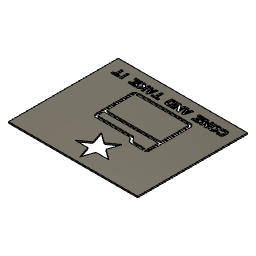
ComeAndTakeIt (Autodesk Fusion 360 design; units mm, degrees)
Autodesk Fusion 360 part; units mm, degrees
(part 1 of 2)
sketch "Sketch1" plane through (0, 0, 0) normal (0, 1, 0) x (1, 0, 0)
  line L0 (0, 0) -> (140, 0)
  line L1 (140, 0) -> (140, -85)
  line L2 (140, -85) -> (0, -85)
  line L3 (0, -85) -> (0, 0)
  constraint horizontal L0
  constraint vertical L1
  constraint horizontal L2
  constraint vertical L3
  constraint coincident L0.start L3.end
extrude "Extrude1" add sketch "Sketch1" along normal blind 2
sketch "Sketch2" plane through (0, 2, 0) normal (0, 1, 0) x (-1, 0, 0)
  line L0 (0, 85) -> (-140, 85)
  line L1 (-140, 85) -> (-140, 0)
  line L2 (-140, 0) -> (0, 0)
  line L3 (0, 0) -> (0, 85)
  spline S0 degree 3 poles (-116.9301, 6.5861) (-117.7721, 6.8255) (-117.8476, 7.0711) (-117.8471, 9.57) knots 0 0 0 0 1 1 1 1
  spline S1 degree 3 poles (-117.8471, 9.57) (-117.8467, 12.3494) (-117.7458, 12.5338) (-116.1845, 12.6085) knots 0 0 0 0 1 1 1 1
  line L4 (-116.1845, 12.6085) -> (-115.3705, 12.6474)
  line L5 (-115.3705, 12.6474) -> (-115.3705, 11.8564)
  line L6 (-115.3705, 11.8564) -> (-115.3705, 11.0653)
  line L7 (-115.3705, 11.0653) -> (-115.8292, 11.0653)
  line L8 (-115.8292, 11.0653) -> (-116.2879, 11.0653)
  line L9 (-116.2879, 11.0653) -> (-116.2879, 9.5516)
  line L10 (-116.2879, 9.5516) -> (-116.2879, 8.0379)
  line L11 (-116.2879, 8.0379) -> (-115.8292, 8.0379)
  line L12 (-115.8292, 8.0379) -> (-115.3705, 8.0379)
  line L13 (-115.3705, 8.0379) -> (-115.3705, 7.2581)
  line L14 (-115.3705, 7.2581) -> (-115.3705, 6.4783)
  line L15 (-115.3705, 6.4783) -> (-115.9897, 6.4865)
  spline S2 degree 3 poles (-115.9897, 6.4865) (-116.3303, 6.4911) (-116.7535, 6.5359) (-116.9301, 6.5861) knots 0 0 0 0 1 1 1 1
  line L16 (-115.0035, 7.2486) -> (-115.0035, 8.0379)
  line L17 (-115.0035, 8.0379) -> (-114.5448, 8.0379)
  spline S3 degree 3 poles (-114.5448, 8.0379) (-114.1167, 8.0379) (-114.0861, 8.0532) (-114.0861, 8.2672) knots 0 0 0 0 1 1 1 1
  spline S4 degree 3 poles (-114.0861, 8.2672) (-114.0861, 8.4941) (-114.0776, 8.4966) (-113.2956, 8.4966) knots 0 0 0 0 1 1 1 1
  line L18 (-113.2956, 8.4966) -> (-112.5051, 8.4966)
  line L19 (-112.5051, 8.4966) -> (-112.543, 7.9012)
  spline S5 degree 3 poles (-112.543, 7.9012) (-112.6079, 6.8826) (-113.0093, 6.551) (-114.2466, 6.4942) knots 0 0 0 0 1 1 1 1
  line L20 (-114.2466, 6.4942) -> (-115.0035, 6.4594)
  line L21 (-115.0035, 6.4594) -> (-115.0035, 7.2486)
  spline S6 degree 3 poles (-110.7834, 6.5861) (-111.6154, 6.8226) (-111.7009, 7.1053) (-111.7005, 9.6175) knots 0 0 0 0 1 1 1 1
  spline S7 degree 3 poles (-111.7005, 9.6175) (-111.7, 12.3429) (-111.5937, 12.5341) (-110.0378, 12.6085) knots 0 0 0 0 1 1 1 1
  line L22 (-110.0378, 12.6085) -> (-109.2238, 12.6474)
  line L23 (-109.2238, 12.6474) -> (-109.2238, 11.8564)
  line L24 (-109.2238, 11.8564) -> (-109.2238, 11.0653)
  line L25 (-109.2238, 11.0653) -> (-109.6825, 11.0653)
  line L26 (-109.6825, 11.0653) -> (-110.1412, 11.0653)
  line L27 (-110.1412, 11.0653) -> (-110.1412, 9.5516)
  line L28 (-110.1412, 9.5516) -> (-110.1412, 8.0379)
  line L29 (-110.1412, 8.0379) -> (-109.6825, 8.0379)
  line L30 (-109.6825, 8.0379) -> (-109.2238, 8.0379)
  line L31 (-109.2238, 8.0379) -> (-109.2238, 7.2581)
  line L32 (-109.2238, 7.2581) -> (-109.2238, 6.4783)
  line L33 (-109.2238, 6.4783) -> (-109.843, 6.4865)
  spline S8 degree 3 poles (-109.843, 6.4865) (-110.1836, 6.4911) (-110.6068, 6.5359) (-110.7834, 6.5861) knots 0 0 0 0 1 1 1 1
  line L34 (-108.8568, 7.2486) -> (-108.8568, 8.0379)
  line L35 (-108.8568, 8.0379) -> (-108.3981, 8.0379)
  line L36 (-108.3981, 8.0379) -> (-107.9394, 8.0379)
  line L37 (-107.9394, 8.0379) -> (-107.9394, 9.5516)
  line L38 (-107.9394, 9.5516) -> (-107.9394, 11.0653)
  line L39 (-107.9394, 11.0653) -> (-108.3981, 11.0653)
  line L40 (-108.3981, 11.0653) -> (-108.8568, 11.0653)
  line L41 (-108.8568, 11.0653) -> (-108.8568, 11.8543)
  line L42 (-108.8568, 11.8543) -> (-108.8568, 12.6432)
  line L43 (-108.8568, 12.6432) -> (-108.0377, 12.6111)
  spline S9 degree 3 poles (-108.0377, 12.6111) (-106.4829, 12.5503) (-106.366, 12.3243) (-106.4003, 9.4434) knots 0 0 0 0 1 1 1 1
  spline S10 degree 3 poles (-106.4003, 9.4434) (-106.4329, 6.7089) (-106.5146, 6.567) (-108.0999, 6.4942) knots 0 0 0 0 1 1 1 1
  line L44 (-108.0999, 6.4942) -> (-108.8568, 6.4594)
  line L45 (-108.8568, 6.4594) -> (-108.8568, 7.2486)
  line L46 (-105.5526, 9.1617) -> (-105.5511, 11.8451)
  line L47 (-105.5511, 11.8451) -> (-104.7728, 10.3571)
  line L48 (-104.7728, 10.3571) -> (-103.9945, 8.869)
  line L49 (-103.9945, 8.869) -> (-103.9945, 7.6736)
  line L50 (-103.9945, 7.6736) -> (-103.9945, 6.4783)
  line L51 (-103.9945, 6.4783) -> (-104.7743, 6.4783)
  line L52 (-104.7743, 6.4783) -> (-105.5541, 6.4783)
  line L53 (-105.5541, 6.4783) -> (-105.5526, 9.1617)
  line L54 (-101.7927, 8.0726) -> (-101.7927, 9.6669)
  line L55 (-101.7927, 9.6669) -> (-102.2055, 10.4133)
  spline S11 degree 3 poles (-102.2055, 10.4133) (-102.7007, 11.3085) (-102.7017, 11.1051) (-102.1987, 11.9336) knots 0 0 0 0 1 1 1 1
  line L56 (-102.1987, 11.9336) -> (-101.779, 12.625)
  line L57 (-101.779, 12.625) -> (-101.006, 12.625)
  line L58 (-101.006, 12.625) -> (-100.2331, 12.625)
  line L59 (-100.2331, 12.625) -> (-100.2331, 9.5516)
  line L60 (-100.2331, 9.5516) -> (-100.2331, 6.4783)
  line L61 (-100.2331, 6.4783) -> (-101.0129, 6.4783)
  line L62 (-101.0129, 6.4783) -> (-101.7927, 6.4783)
  line L63 (-101.7927, 6.4783) -> (-101.7927, 8.0726)
  line L64 (-99.4074, 9.5516) -> (-99.4074, 12.625)
  line L65 (-99.4074, 12.625) -> (-98.6276, 12.625)
  line L66 (-98.6276, 12.625) -> (-97.8478, 12.625)
  line L67 (-97.8478, 12.625) -> (-97.8478, 11.4782)
  line L68 (-97.8478, 11.4782) -> (-97.8478, 10.3314)
  line L69 (-97.8478, 10.3314) -> (-96.701, 10.3314)
  line L70 (-96.701, 10.3314) -> (-95.5543, 10.3314)
  line L71 (-95.5543, 10.3314) -> (-95.5543, 9.5516)
  line L72 (-95.5543, 9.5516) -> (-95.5543, 8.7718)
  line L73 (-95.5543, 8.7718) -> (-96.701, 8.7718)
  line L74 (-96.701, 8.7718) -> (-97.8478, 8.7718)
  line L75 (-97.8478, 8.7718) -> (-97.8478, 7.625)
  line L76 (-97.8478, 7.625) -> (-97.8478, 6.4783)
  line L77 (-97.8478, 6.4783) -> (-98.6276, 6.4783)
  line L78 (-98.6276, 6.4783) -> (-99.4074, 6.4783)
  line L79 (-99.4074, 6.4783) -> (-99.4074, 9.5516)
  spline S12 degree 3 poles (-97.5114, 6.5394) (-97.5451, 6.5731) (-97.5726, 6.924) (-97.5726, 7.3192) knots 0 0 0 0 1 1 1 1
  line L80 (-97.5726, 7.3192) -> (-97.5726, 8.0379)
  line L81 (-97.5726, 8.0379) -> (-95.8295, 8.0379)
  line L82 (-95.8295, 8.0379) -> (-94.0864, 8.0379)
  line L83 (-94.0864, 8.0379) -> (-94.0864, 7.2581)
  line L84 (-94.0864, 7.2581) -> (-94.0864, 6.4783)
  line L85 (-94.0864, 6.4783) -> (-95.7683, 6.4783)
  spline S13 degree 3 poles (-95.7683, 6.4783) (-96.6934, 6.4783) (-97.4778, 6.5058) (-97.5114, 6.5394) knots 0 0 0 0 1 1 1 1
  spline S14 degree 3 poles (-89.9398, 6.5892) (-89.9175, 6.6543) (-89.5512, 7.8319) (-89.1259, 9.206) knots 0 0 0 0 1 1 1 1
  spline S15 degree 3 poles (-89.1259, 9.206) (-88.7005, 10.5801) (-88.3319, 11.7045) (-88.3067, 11.7047) knots 0 0 0 0 1 1 1 1
  spline S16 degree 3 poles (-88.3067, 11.7047) (-88.2815, 11.7049) (-88.0086, 10.8489) (-87.7004, 9.8026) knots 0 0 0 0 1 1 1 1
  line L86 (-87.7004, 9.8026) -> (-87.14, 7.9003)
  line L87 (-87.14, 7.9003) -> (-87.5603, 7.8544)
  line L88 (-87.5603, 7.8544) -> (-87.9805, 7.8085)
  line L89 (-87.9805, 7.8085) -> (-88.1725, 7.1663)
  line L90 (-88.1725, 7.1663) -> (-88.3645, 6.5241)
  line L91 (-88.3645, 6.5241) -> (-89.1725, 6.4975)
  spline S17 degree 3 poles (-89.1725, 6.4975) (-89.8011, 6.4767) (-89.9715, 6.4971) (-89.9398, 6.5892) knots 0 0 0 0 1 1 1 1
  spline S18 degree 3 poles (-87.0995, 9.4403) (-88.2214, 13.0061) (-88.201, 12.625) (-87.2699, 12.625) knots 0 0 0 0 1 1 1 1
  line L92 (-87.2699, 12.625) -> (-86.5083, 12.625)
  line L93 (-86.5083, 12.625) -> (-85.5727, 9.6479)
  spline S19 degree 3 poles (-85.5727, 9.6479) (-85.0581, 8.0104) (-84.637, 6.6274) (-84.637, 6.5745) knots 0 0 0 0 1 1 1 1
  spline S20 degree 3 poles (-84.637, 6.5745) (-84.637, 6.515) (-84.9294, 6.4783) (-85.4023, 6.4783) knots 0 0 0 0 1 1 1 1
  line L94 (-85.4023, 6.4783) -> (-86.1675, 6.4783)
  line L95 (-86.1675, 6.4783) -> (-87.0995, 9.4403)
  spline S21 degree 3 poles (-84.1783, 8.7718) (-84.1783, 10.0333) (-84.16, 11.0653) (-84.1377, 11.0653) knots 0 0 0 0 1 1 1 1
  spline S22 degree 3 poles (-84.1377, 11.0653) (-84.1153, 11.0653) (-83.7644, 10.6018) (-83.3579, 10.0354) knots 0 0 0 0 1 1 1 1
  line L96 (-83.3579, 10.0354) -> (-82.6187, 9.0054)
  line L97 (-82.6187, 9.0054) -> (-82.6187, 7.7418)
  line L98 (-82.6187, 7.7418) -> (-82.6187, 6.4783)
  line L99 (-82.6187, 6.4783) -> (-83.3985, 6.4783)
  line L100 (-83.3985, 6.4783) -> (-84.1783, 6.4783)
  line L101 (-84.1783, 6.4783) -> (-84.1783, 8.7718)
  spline S23 degree 3 poles (-82.2755, 9.1431) (-84.0735, 11.6611) (-84.1783, 11.8307) (-84.1783, 12.22) knots 0 0 0 0 1 1 1 1
  line L102 (-84.1783, 12.22) -> (-84.1783, 12.6321)
  line L103 (-84.1783, 12.6321) -> (-83.3779, 12.6056)
  line L104 (-83.3779, 12.6056) -> (-82.5774, 12.5791)
  line L105 (-82.5774, 12.5791) -> (-80.7274, 9.9771)
  spline S24 degree 3 poles (-80.7274, 9.9771) (-78.3715, 6.6635) (-78.3129, 6.4783) (-79.6205, 6.4783) knots 0 0 0 0 1 1 1 1
  line L106 (-79.6205, 6.4783) -> (-80.3728, 6.4783)
  line L107 (-80.3728, 6.4783) -> (-82.2755, 9.1431)
  line L108 (-78.0316, 9.5516) -> (-78.0316, 12.625)
  line L109 (-78.0316, 12.625) -> (-77.2518, 12.625)
  line L110 (-77.2518, 12.625) -> (-76.472, 12.625)
  line L111 (-76.472, 12.625) -> (-76.472, 9.5516)
  line L112 (-76.472, 9.5516) -> (-76.472, 6.4783)
  line L113 (-76.472, 6.4783) -> (-77.2518, 6.4783)
  line L114 (-77.2518, 6.4783) -> (-78.0316, 6.4783)
  line L115 (-78.0316, 6.4783) -> (-78.0316, 9.5516)
  line L116 (-76.105, 7.251) -> (-76.105, 8.0379)
  line L117 (-76.105, 8.0379) -> (-75.1876, 8.0379)
  line L118 (-75.1876, 8.0379) -> (-74.2702, 8.0379)
  line L119 (-74.2702, 8.0379) -> (-74.2702, 9.5516)
  line L120 (-74.2702, 9.5516) -> (-74.2702, 11.0653)
  line L121 (-74.2702, 11.0653) -> (-75.1876, 11.0653)
  line L122 (-75.1876, 11.0653) -> (-76.105, 11.0653)
  line L123 (-76.105, 11.0653) -> (-76.105, 11.8452)
  line L124 (-76.105, 11.8452) -> (-76.105, 12.625)
  line L125 (-76.105, 12.625) -> (-74.9553, 12.625)
  spline S25 degree 3 poles (-74.9553, 12.625) (-73.6992, 12.625) (-73.3704, 12.5415) (-72.9858, 12.125) knots 0 0 0 0 1 1 1 1
  line L126 (-72.9858, 12.125) -> (-72.7565, 11.8766)
  line L127 (-72.7565, 11.8766) -> (-72.7291, 9.6563)
  spline S26 degree 3 poles (-72.7291, 9.6563) (-72.6916, 6.6133) (-72.7367, 6.5473) (-74.8895, 6.4941) knots 0 0 0 0 1 1 1 1
  line L128 (-74.8895, 6.4941) -> (-76.105, 6.4641)
  line L129 (-76.105, 6.4641) -> (-76.105, 7.251)
  line L130 (-66.197, 9.5516) -> (-66.197, 12.625)
  line L131 (-66.197, 12.625) -> (-65.4172, 12.625)
  line L132 (-65.4172, 12.625) -> (-64.6373, 12.625)
  line L133 (-64.6373, 12.625) -> (-64.6373, 9.5516)
  line L134 (-64.6373, 9.5516) -> (-64.6373, 6.4783)
  line L135 (-64.6373, 6.4783) -> (-65.4172, 6.4783)
  line L136 (-65.4172, 6.4783) -> (-66.197, 6.4783)
  line L137 (-66.197, 6.4783) -> (-66.197, 9.5516)
  spline S27 degree 3 poles (-62.4093, 6.5979) (-62.3824, 6.6679) (-62.0205, 7.8152) (-61.6049, 9.1475) knots 0 0 0 0 1 1 1 1
  spline S28 degree 3 poles (-61.6049, 9.1475) (-61.1894, 10.4798) (-60.8211, 11.6021) (-60.7866, 11.6414) knots 0 0 0 0 1 1 1 1
  spline S29 degree 3 poles (-60.7866, 11.6414) (-60.7521, 11.6807) (-60.484, 10.8963) (-60.191, 9.8983) knots 0 0 0 0 1 1 1 1
  spline S30 degree 3 poles (-60.191, 9.8983) (-59.8979, 8.9003) (-59.6387, 8.0321) (-59.615, 7.9691) knots 0 0 0 0 1 1 1 1
  spline S31 degree 3 poles (-59.615, 7.9691) (-59.5845, 7.8879) (-59.6931, 7.8544) (-59.9869, 7.8544) knots 0 0 0 0 1 1 1 1
  line L138 (-59.9869, 7.8544) -> (-60.4019, 7.8544)
  line L139 (-60.4019, 7.8544) -> (-60.6234, 7.1893)
  line L140 (-60.6234, 7.1893) -> (-60.8449, 6.5241)
  line L141 (-60.8449, 6.5241) -> (-61.6515, 6.4975)
  spline S32 degree 3 poles (-61.6515, 6.4975) (-62.3087, 6.4757) (-62.449, 6.4943) (-62.4093, 6.5979) knots 0 0 0 0 1 1 1 1
  line L142 (-62.4093, 6.5979) -> (-62.4093, 6.5979)
  spline S33 degree 3 poles (-59.5715, 9.4828) (-60.0876, 11.1353) (-60.5097, 12.5183) (-60.5094, 12.5561) knots 0 0 0 0 1 1 1 1
  spline S34 degree 3 poles (-60.5094, 12.5561) (-60.5094, 12.594) (-60.1613, 12.625) (-59.7363, 12.625) knots 0 0 0 0 1 1 1 1
  line L143 (-59.7363, 12.625) -> (-58.9636, 12.625)
  line L144 (-58.9636, 12.625) -> (-58.8693, 12.3268)
  spline S35 degree 3 poles (-58.8693, 12.3268) (-56.7969, 5.7737) (-56.9168, 6.4783) (-57.8738, 6.4783) knots 0 0 0 0 1 1 1 1
  line L145 (-57.8738, 6.4783) -> (-58.6331, 6.4783)
  line L146 (-58.6331, 6.4783) -> (-59.5715, 9.4828)
  line L147 (-56.6558, 9.5516) -> (-56.6558, 12.625)
  line L148 (-56.6558, 12.625) -> (-55.876, 12.625)
  line L149 (-55.876, 12.625) -> (-55.0962, 12.625)
  line L150 (-55.0962, 12.625) -> (-55.0962, 9.5516)
  line L151 (-55.0962, 9.5516) -> (-55.0962, 6.4783)
  line L152 (-55.0962, 6.4783) -> (-55.876, 6.4783)
  line L153 (-55.876, 6.4783) -> (-56.6558, 6.4783)
  line L154 (-56.6558, 6.4783) -> (-56.6558, 9.5516)
  line L155 (-53.7889, 7.6168) -> (-54.7293, 8.7561)
  line L156 (-54.7293, 8.7561) -> (-54.7271, 9.5667)
  line L157 (-54.7271, 9.5667) -> (-54.7249, 10.3773)
  line L158 (-54.7249, 10.3773) -> (-53.7899, 11.5011)
  line L159 (-53.7899, 11.5011) -> (-52.8549, 12.6249)
  line L160 (-52.8549, 12.6249) -> (-52.049, 12.6249)
  line L161 (-52.049, 12.6249) -> (-51.2431, 12.6249)
  line L162 (-51.2431, 12.6249) -> (-51.2431, 12.2337)
  spline S36 degree 3 poles (-51.2431, 12.2337) (-51.2431, 11.855) (-51.2801, 11.8055) (-52.3899, 10.6983) knots 0 0 0 0 1 1 1 1
  line L163 (-52.3899, 10.6983) -> (-53.5367, 9.5543)
  line L164 (-53.5367, 9.5543) -> (-52.3835, 8.3984)
  spline S37 degree 3 poles (-52.3835, 8.3984) (-51.2611, 7.2735) (-51.231, 7.233) (-51.2596, 6.8834) knots 0 0 0 0 1 1 1 1
  line L165 (-51.2596, 6.8834) -> (-51.289, 6.5241)
  line L166 (-51.289, 6.5241) -> (-52.0688, 6.5008)
  line L167 (-52.0688, 6.5008) -> (-52.8486, 6.4775)
  line L168 (-52.8486, 6.4775) -> (-53.7889, 7.6168)
  line L169 (-50.5091, 9.5516) -> (-50.5091, 12.625)
  line L170 (-50.5091, 12.625) -> (-49.7293, 12.625)
  line L171 (-49.7293, 12.625) -> (-48.9495, 12.625)
  line L172 (-48.9495, 12.625) -> (-48.9495, 11.4782)
  line L173 (-48.9495, 11.4782) -> (-48.9495, 10.3314)
  line L174 (-48.9495, 10.3314) -> (-47.8028, 10.3314)
  line L175 (-47.8028, 10.3314) -> (-46.656, 10.3314)
  line L176 (-46.656, 10.3314) -> (-46.656, 9.5516)
  line L177 (-46.656, 9.5516) -> (-46.656, 8.7718)
  line L178 (-46.656, 8.7718) -> (-47.8028, 8.7718)
  line L179 (-47.8028, 8.7718) -> (-48.9495, 8.7718)
  line L180 (-48.9495, 8.7718) -> (-48.9495, 7.625)
  line L181 (-48.9495, 7.625) -> (-48.9495, 6.4783)
  line L182 (-48.9495, 6.4783) -> (-49.7293, 6.4783)
  line L183 (-49.7293, 6.4783) -> (-50.5091, 6.4783)
  line L184 (-50.5091, 6.4783) -> (-50.5091, 9.5516)
  line L185 (-48.5826, 7.2581) -> (-48.5826, 8.0379)
  line L186 (-48.5826, 8.0379) -> (-46.8395, 8.0379)
  line L187 (-46.8395, 8.0379) -> (-45.0964, 8.0379)
  line L188 (-45.0964, 8.0379) -> (-45.0964, 7.2581)
  line L189 (-45.0964, 7.2581) -> (-45.0964, 6.4783)
  line L190 (-45.0964, 6.4783) -> (-46.8395, 6.4783)
  line L191 (-46.8395, 6.4783) -> (-48.5826, 6.4783)
  line L192 (-48.5826, 6.4783) -> (-48.5826, 7.2581)
  line L193 (-40.0506, 9.5516) -> (-40.0506, 12.625)
  line L194 (-40.0506, 12.625) -> (-39.2708, 12.625)
  line L195 (-39.2708, 12.625) -> (-38.491, 12.625)
  line L196 (-38.491, 12.625) -> (-38.491, 9.5516)
  line L197 (-38.491, 9.5516) -> (-38.491, 6.4783)
  line L198 (-38.491, 6.4783) -> (-39.2708, 6.4783)
  line L199 (-39.2708, 6.4783) -> (-40.0506, 6.4783)
  line L200 (-40.0506, 6.4783) -> (-40.0506, 9.5516)
  line L201 (-35.4635, 9.5516) -> (-35.4635, 12.625)
  line L202 (-35.4635, 12.625) -> (-34.6837, 12.625)
  line L203 (-34.6837, 12.625) -> (-33.9039, 12.625)
  line L204 (-33.9039, 12.625) -> (-33.9039, 9.5516)
  line L205 (-33.9039, 9.5516) -> (-33.9039, 6.4783)
  line L206 (-33.9039, 6.4783) -> (-34.6837, 6.4783)
  line L207 (-34.6837, 6.4783) -> (-35.4635, 6.4783)
  line L208 (-35.4635, 6.4783) -> (-35.4635, 9.5516)
  spline S38 degree 3 poles (-104.2491, 10.0989) (-104.9669, 11.4344) (-105.5541, 12.549) (-105.5541, 12.576) knots 0 0 0 0 1 1 1 1
  spline S39 degree 3 poles (-105.5541, 12.576) (-105.5541, 12.6029) (-105.2075, 12.6249) (-104.7839, 12.6249) knots 0 0 0 0 1 1 1 1
  line L209 (-104.7839, 12.6249) -> (-104.0137, 12.6249)
  line L210 (-104.0137, 12.6249) -> (-103.0464, 10.9781)
  line L211 (-103.0464, 10.9781) -> (-102.0791, 9.3313)
  line L212 (-102.0791, 9.3313) -> (-102.4626, 8.5011)
  spline S40 degree 3 poles (-102.4626, 8.5011) (-102.9419, 7.4634) (-102.7314, 7.2751) (-104.2491, 10.0989) knots 0 0 0 0 1 1 1 1
  line L213 (-79.66, 9.1105) -> (-80.4169, 10.1795)
  line L214 (-80.4169, 10.1795) -> (-80.4169, 11.4022)
  line L215 (-80.4169, 11.4022) -> (-80.4169, 12.6249)
  line L216 (-80.4169, 12.6249) -> (-79.6371, 12.6249)
  line L217 (-79.6371, 12.6249) -> (-78.8573, 12.6249)
  line L218 (-78.8573, 12.6249) -> (-78.8573, 10.3314)
  spline S41 degree 3 poles (-78.8573, 10.3314) (-78.8573, 9.07) (-78.8676, 8.0387) (-78.8802, 8.0397) knots 0 0 0 0 1 1 1 1
  spline S42 degree 3 poles (-78.8802, 8.0397) (-78.8928, 8.0407) (-79.2438, 8.5225) (-79.66, 9.1105) knots 0 0 0 0 1 1 1 1
  spline S43 degree 3 poles (-114.0861, 10.8819) (-114.0861, 11.0409) (-114.1472, 11.0653) (-114.5448, 11.0653) knots 0 0 0 0 1 1 1 1
  line L219 (-114.5448, 11.0653) -> (-115.0035, 11.0653)
  line L220 (-115.0035, 11.0653) -> (-115.0035, 11.8451)
  line L221 (-115.0035, 11.8451) -> (-115.0035, 12.6249)
  line L222 (-115.0035, 12.6249) -> (-114.2925, 12.6247)
  spline S44 degree 3 poles (-114.2925, 12.6247) (-113.1069, 12.6245) (-112.6158, 12.2383) (-112.5443, 11.25) knots 0 0 0 0 1 1 1 1
  line L223 (-112.5443, 11.25) -> (-112.5044, 10.6983)
  line L224 (-112.5044, 10.6983) -> (-113.2953, 10.6983)
  spline S45 degree 3 poles (-113.2953, 10.6983) (-114.0249, 10.6983) (-114.0861, 10.7125) (-114.0861, 10.8818) knots 0 0 0 0 1 1 1 1
  line L225 (-114.0861, 10.8818) -> (-114.0861, 10.8819)
  line L226 (-97.5726, 11.8451) -> (-97.5726, 12.6249)
  line L227 (-97.5726, 12.6249) -> (-95.8295, 12.6249)
  line L228 (-95.8295, 12.6249) -> (-94.0864, 12.6249)
  line L229 (-94.0864, 12.6249) -> (-94.0864, 11.8451)
  line L230 (-94.0864, 11.8451) -> (-94.0864, 11.0653)
  line L231 (-94.0864, 11.0653) -> (-95.8295, 11.0653)
  line L232 (-95.8295, 11.0653) -> (-97.5726, 11.0653)
  line L233 (-97.5726, 11.0653) -> (-97.5726, 11.8451)
  line L234 (-68.1235, 11.8451) -> (-68.1235, 12.6249)
  line L235 (-68.1235, 12.6249) -> (-67.2979, 12.6249)
  line L236 (-67.2979, 12.6249) -> (-66.4722, 12.6249)
  line L237 (-66.4722, 12.6249) -> (-66.4722, 11.8451)
  line L238 (-66.4722, 11.8451) -> (-66.4722, 11.0653)
  line L239 (-66.4722, 11.0653) -> (-67.2979, 11.0653)
  line L240 (-67.2979, 11.0653) -> (-68.1235, 11.0653)
  line L241 (-68.1235, 11.0653) -> (-68.1235, 11.8451)
  line L242 (-64.2704, 11.8451) -> (-64.2704, 12.6249)
  line L243 (-64.2704, 12.6249) -> (-63.4906, 12.6249)
  line L244 (-63.4906, 12.6249) -> (-62.7108, 12.6249)
  line L245 (-62.7108, 12.6249) -> (-62.7108, 11.8451)
  line L246 (-62.7108, 11.8451) -> (-62.7108, 11.0653)
  line L247 (-62.7108, 11.0653) -> (-63.4906, 11.0653)
  line L248 (-63.4906, 11.0653) -> (-64.2704, 11.0653)
  line L249 (-64.2704, 11.0653) -> (-64.2704, 11.8451)
  line L250 (-48.5826, 11.8451) -> (-48.5826, 12.6249)
  line L251 (-48.5826, 12.6249) -> (-46.8395, 12.6249)
  line L252 (-46.8395, 12.6249) -> (-45.0964, 12.6249)
  line L253 (-45.0964, 12.6249) -> (-45.0964, 11.8451)
  line L254 (-45.0964, 11.8451) -> (-45.0964, 11.0653)
  line L255 (-45.0964, 11.0653) -> (-46.8395, 11.0653)
  line L256 (-46.8395, 11.0653) -> (-48.5826, 11.0653)
  line L257 (-48.5826, 11.0653) -> (-48.5826, 11.8451)
  line L258 (-37.2983, 11.8451) -> (-37.2983, 12.6249)
  line L259 (-37.2983, 12.6249) -> (-36.5185, 12.6249)
  line L260 (-36.5185, 12.6249) -> (-35.7387, 12.6249)
  line L261 (-35.7387, 12.6249) -> (-35.7387, 11.8451)
  line L262 (-35.7387, 11.8451) -> (-35.7387, 11.0653)
  line L263 (-35.7387, 11.0653) -> (-36.5185, 11.0653)
  line L264 (-36.5185, 11.0653) -> (-37.2983, 11.0653)
  line L265 (-37.2983, 11.0653) -> (-37.2983, 11.8451)
  line L266 (-33.5369, 11.8451) -> (-33.5369, 12.6249)
  line L267 (-33.5369, 12.6249) -> (-32.7571, 12.6249)
  line L268 (-32.7571, 12.6249) -> (-31.9773, 12.6249)
  line L269 (-31.9773, 12.6249) -> (-31.9773, 11.8451)
  line L270 (-31.9773, 11.8451) -> (-31.9773, 11.0653)
  line L271 (-31.9773, 11.0653) -> (-32.7571, 11.0653)
  line L272 (-32.7571, 11.0653) -> (-33.5369, 11.0653)
  line L273 (-33.5369, 11.0653) -> (-33.5369, 11.8451)
  line L274 (-89.4076, 15.6509) -> (-97.3432, 15.6983)
  line L275 (-97.3432, 15.6983) -> (-97.7592, 15.9429)
  spline S46 degree 3 poles (-97.7592, 15.9429) (-98.3332, 16.2803) (-99.0048, 17.0223) (-99.1226, 17.4492) knots 0 0 0 0 1 1 1 1
  spline S47 degree 3 poles (-99.1226, 17.4492) (-99.4444, 18.6147) (-99.3148, 50.4081) (-98.9864, 50.8517) knots 0 0 0 0 1 1 1 1
  spline S48 degree 3 poles (-98.9864, 50.8517) (-98.7201, 51.2114) (-97.9878, 51.753) (-97.6115, 51.8685) knots 0 0 0 0 1 1 1 1
  line L276 (-97.6115, 51.8685) -> (-97.2974, 51.9649)
  line L277 (-97.2974, 51.9649) -> (-97.2974, 46.6984)
  line L278 (-97.2974, 46.6984) -> (-97.2974, 41.4318)
  line L279 (-97.2974, 41.4318) -> (-76.2784, 41.4318)
  line L280 (-76.2784, 41.4318) -> (-55.2594, 41.4318)
  line L281 (-55.2594, 41.4318) -> (-55.293, 43.7621)
  spline S49 degree 3 poles (-55.293, 43.7621) (-55.3226, 45.8252) (-55.3449, 46.1127) (-55.4873, 46.2701) knots 0 0 0 0 1 1 1 1
  spline S50 degree 3 poles (-55.4873, 46.2701) (-55.6446, 46.4439) (-55.9559, 46.4493) (-69.4629, 46.5127) knots 0 0 0 0 1 1 1 1
  line L282 (-69.4629, 46.5127) -> (-83.2775, 46.5775)
  line L283 (-83.2775, 46.5775) -> (-83.6132, 46.7899)
  spline S51 degree 3 poles (-83.6132, 46.7899) (-84.0925, 47.093) (-84.5925, 47.6658) (-85.3491, 48.778) knots 0 0 0 0 1 1 1 1
  spline S52 degree 3 poles (-85.3491, 48.778) (-86.3565, 50.2589) (-85.6436, 50.0899) (-91.0655, 50.1326) knots 0 0 0 0 1 1 1 1
  line L284 (-91.0655, 50.1326) -> (-95.7377, 50.1693)
  line L285 (-95.7377, 50.1693) -> (-95.7377, 51.1246)
  line L286 (-95.7377, 51.1246) -> (-95.7377, 52.0799)
  line L287 (-95.7377, 52.0799) -> (-90.8066, 52.0539)
  spline S53 degree 3 poles (-90.8066, 52.0539) (-84.8327, 52.0225) (-85.4154, 52.1981) (-83.8295, 49.9505) knots 0 0 0 0 1 1 1 1
  spline S54 degree 3 poles (-83.8295, 49.9505) (-83.4253, 49.3775) (-82.9842, 48.8055) (-82.8493, 48.6794) knots 0 0 0 0 1 1 1 1
  line L288 (-82.8493, 48.6794) -> (-82.604, 48.45)
  line L289 (-82.604, 48.45) -> (-69.0565, 48.4042)
  line L290 (-69.0565, 48.4042) -> (-55.5091, 48.3583)
  line L291 (-55.5091, 48.3583) -> (-55.1061, 48.1434)
  spline S55 degree 3 poles (-55.1061, 48.1434) (-54.6208, 47.8845) (-53.8458, 47.1763) (-53.6648, 46.8263) knots 0 0 0 0 1 1 1 1
  spline S56 degree 3 poles (-53.6648, 46.8263) (-53.3753, 46.2666) (-53.3465, 44.7233) (-53.3728, 31.2026) knots 0 0 0 0 1 1 1 1
  line L292 (-53.3728, 31.2026) -> (-53.399, 17.7166)
  line L293 (-53.399, 17.7166) -> (-53.596, 17.3496)
  spline S57 degree 3 poles (-53.596, 17.3496) (-53.8795, 16.8215) (-54.464, 16.1895) (-54.8891, 15.9513) knots 0 0 0 0 1 1 1 1
  line L294 (-54.8891, 15.9513) -> (-55.2563, 15.7456)
  line L295 (-55.2563, 15.7456) -> (-55.2956, 27.4879)
  spline S58 degree 3 poles (-55.2956, 27.4879) (-55.3251, 36.2918) (-55.3618, 39.257) (-55.4423, 39.3376) knots 0 0 0 0 1 1 1 1
  spline S59 degree 3 poles (-55.4423, 39.3376) (-55.8111, 39.7064) (-96.7705, 39.7018) (-97.1394, 39.3329) knots 0 0 0 0 1 1 1 1
  spline S60 degree 3 poles (-97.1394, 39.3329) (-97.3502, 39.1222) (-97.297, 17.8727) (-97.0853, 17.7179) knots 0 0 0 0 1 1 1 1
  spline S61 degree 3 poles (-97.0853, 17.7179) (-96.7708, 17.4879) (-94.8435, 17.4684) (-75.6693, 17.5007) knots 0 0 0 0 1 1 1 1
  line L296 (-75.6693, 17.5007) -> (-56.4723, 17.5331)
  line L297 (-56.4723, 17.5331) -> (-56.4723, 16.5469)
  line L298 (-56.4723, 16.5469) -> (-56.4723, 15.5607)
  line L299 (-56.4723, 15.5607) -> (-68.9721, 15.5821)
  spline S62 degree 3 poles (-68.9721, 15.5821) (-75.847, 15.5939) (-85.043, 15.6249) (-89.4076, 15.6509) knots 0 0 0 0 1 1 1 1
  spline S63 degree 3 poles (-84.2701, 56.5783) (-84.2701, 56.6337) (-83.6739, 58.5224) (-82.9452, 60.7754) knots 0 0 0 0 1 1 1 1
  spline S64 degree 3 poles (-82.9452, 60.7754) (-82.2166, 63.0284) (-81.5598, 65.0833) (-81.4857, 65.3419) knots 0 0 0 0 1 1 1 1
  line L300 (-81.4857, 65.3419) -> (-81.3511, 65.812)
  line L301 (-81.3511, 65.812) -> (-83.2605, 67.2226)
  spline S65 degree 3 poles (-83.2605, 67.2226) (-84.3107, 67.9984) (-86.0398, 69.2731) (-87.1031, 70.0552) knots 0 0 0 0 1 1 1 1
  spline S66 degree 3 poles (-87.1031, 70.0552) (-88.1663, 70.8373) (-89.0372, 71.5019) (-89.0384, 71.5321) knots 0 0 0 0 1 1 1 1
  spline S67 degree 3 poles (-89.0384, 71.5321) (-89.0428, 71.6427) (-86.9963, 71.7066) (-83.4072, 71.7078) knots 0 0 0 0 1 1 1 1
  spline S68 degree 3 poles (-83.4072, 71.7078) (-81.3841, 71.7085) (-79.6443, 71.7318) (-79.541, 71.7595) knots 0 0 0 0 1 1 1 1
  spline S69 degree 3 poles (-79.541, 71.7595) (-79.3833, 71.8019) (-79.1228, 72.5119) (-77.9172, 76.1848) knots 0 0 0 0 1 1 1 1
  spline S70 degree 3 poles (-77.9172, 76.1848) (-76.6174, 80.1449) (-76.2921, 81.0206) (-76.1729, 80.8806) knots 0 0 0 0 1 1 1 1
  spline S71 degree 3 poles (-76.1729, 80.8806) (-76.1515, 80.8554) (-75.9206, 80.1537) (-75.6599, 79.3211) knots 0 0 0 0 1 1 1 1
  spline S72 degree 3 poles (-75.6599, 79.3211) (-75.3991, 78.4885) (-74.7406, 76.445) (-74.1964, 74.7799) knots 0 0 0 0 1 1 1 1
  line L302 (-74.1964, 74.7799) -> (-73.207, 71.7524)
  line L303 (-73.207, 71.7524) -> (-68.3792, 71.7064)
  spline S73 degree 3 poles (-68.3792, 71.7064) (-65.724, 71.6811) (-63.523, 71.632) (-63.4883, 71.5973) knots 0 0 0 0 1 1 1 1
  spline S74 degree 3 poles (-63.4883, 71.5973) (-63.4536, 71.5626) (-63.8374, 71.2323) (-64.3411, 70.8635) knots 0 0 0 0 1 1 1 1
  spline S75 degree 3 poles (-64.3411, 70.8635) (-64.8448, 70.4946) (-66.5884, 69.2226) (-68.2156, 68.0369) knots 0 0 0 0 1 1 1 1
  spline S76 degree 3 poles (-68.2156, 68.0369) (-69.8429, 66.8511) (-71.1935, 65.8307) (-71.2171, 65.7693) knots 0 0 0 0 1 1 1 1
  spline S77 degree 3 poles (-71.2171, 65.7693) (-71.2407, 65.7079) (-70.8873, 64.5313) (-70.4316, 63.1547) knots 0 0 0 0 1 1 1 1
  spline S78 degree 3 poles (-70.4316, 63.1547) (-69.3764, 59.9665) (-68.4402, 57.0576) (-68.36, 56.7181) knots 0 0 0 0 1 1 1 1
  spline S79 degree 3 poles (-68.36, 56.7181) (-68.267, 56.3244) (-68.2463, 56.311) (-72.3936, 59.3233) knots 0 0 0 0 1 1 1 1
  spline S80 degree 3 poles (-72.3936, 59.3233) (-74.4763, 60.836) (-76.2277, 62.0737) (-76.2858, 62.0737) knots 0 0 0 0 1 1 1 1
  spline S81 degree 3 poles (-76.2858, 62.0737) (-76.3438, 62.0737) (-77.9472, 60.9463) (-79.849, 59.5684) knots 0 0 0 0 1 1 1 1
  spline S82 degree 3 poles (-79.849, 59.5684) (-84.3603, 56.2999) (-84.2701, 56.361) (-84.2701, 56.5783) knots 0 0 0 0 1 1 1 1
extrude "Extrude2" add sketch "Sketch2" along normal blind 4
extrude "Extrude3" cut 1 faces at (46.6667, 0, 28.3333) along direction (0, 1, 0) blind 2
extrude "Extrude4" cut 1 faces at (0, 4.6667, 56.6667) along direction (1, 0, 0) blind 25
extrude "Extrude5" cut 1 faces at (140, 4.6667, 28.3333) along direction (-1, 0, 0) blind 15
extrude "Extrude6" cut 1 faces at (36.8211, 6, 47.8651) along direction (0, -1, 0) blind 2
extrude "Extrude7" cut 1 faces at (36.8493, 4, 48.0613) along direction (0, -1, 0) blind 1
sketch "Sketch3" plane through (0, 3, 0) normal (0, 1, 0) x (-1, 0, 0)
  line L0 (-125, 85) -> (-125, 0)
  line L1 (-125, 0) -> (-25, 0)
  line L2 (-25, 0) -> (-25, 85)
  line L3 (-25, 85) -> (-125, 85)
  line L4 (-76.472, 6.4783) -> (-78.0316, 6.4783)
  line L5 (-78.0316, 6.4783) -> (-78.0316, 9.5516)
  line L6 (-78.0316, 9.5516) -> (-78.0316, 12.625)
  line L7 (-78.0316, 12.625) -> (-76.472, 12.625)
  line L8 (-76.472, 12.625) -> (-76.472, 6.4783)
  line L9 (-66.4722, 11.0653) -> (-68.1235, 11.0653)
  line L10 (-68.1235, 11.0653) -> (-68.1235, 12.6249)
  line L11 (-68.1235, 12.6249) -> (-66.4722, 12.6249)
  line L12 (-66.4722, 12.6249) -> (-66.4722, 11.0653)
  line L13 (-38.491, 6.4783) -> (-40.0506, 6.4783)
  line L14 (-40.0506, 6.4783) -> (-40.0506, 12.625)
  line L15 (-40.0506, 12.625) -> (-38.491, 12.625)
  line L16 (-38.491, 12.625) -> (-38.491, 6.4783)
  line L17 (-52.0688, 6.5008) -> (-52.8486, 6.4775)
  line L18 (-52.8486, 6.4775) -> (-53.7889, 7.6168)
  line L19 (-53.7889, 7.6168) -> (-54.7293, 8.7561)
  line L20 (-54.7293, 8.7561) -> (-54.7249, 10.3773)
  line L21 (-54.7249, 10.3773) -> (-53.7899, 11.5011)
  line L22 (-53.7899, 11.5011) -> (-52.8549, 12.6249)
  line L23 (-52.8549, 12.6249) -> (-51.2431, 12.6249)
  line L24 (-51.2431, 12.6249) -> (-51.2431, 12.2337)
  spline S0 degree 3 poles (-52.3899, 10.6983) (-51.8687, 11.2183) (-51.5805, 11.5083) (-51.354, 11.7976) (-51.3106, 11.8693) (-51.2466, 12.0313) (-51.2431, 12.1168) (-51.2431, 12.2337) knots -0.113831 -0.113831 -0.113831 -0.113831 -0.059792 -0.059792 -0.035054 -0.035054 0 0 0 0
  line L25 (-52.3899, 10.6983) -> (-53.5367, 9.5543)
  line L26 (-53.5367, 9.5543) -> (-52.3835, 8.3984)
  spline S1 degree 3 poles (-51.2596, 6.8834) (-51.2522, 6.9739) (-51.2487, 7.0437) (-51.2843, 7.1852) (-51.3202, 7.2562) (-51.5342, 7.5446) (-51.8221, 7.8358) (-52.3835, 8.3984) knots -0.477393 -0.477393 -0.477393 -0.477393 -0.353588 -0.353588 -0.238442 -0.238442 0 0 0 0
  line L27 (-51.2596, 6.8834) -> (-51.289, 6.5241)
  line L28 (-51.289, 6.5241) -> (-52.0688, 6.5008)
  line L29 (-109.2238, 6.4783) -> (-109.843, 6.4865)
  spline S2 degree 3 poles (-110.7834, 6.5861) (-110.6951, 6.561) (-110.5451, 6.5372) (-110.2047, 6.5012) (-110.0138, 6.4888) (-109.843, 6.4865) knots -0.102601 -0.102601 -0.102601 -0.102601 -0.051232 -0.051232 0 0 0 0
  spline S3 degree 3 poles (-111.7005, 9.6175) (-111.7006, 8.506) (-111.6841, 7.8313) (-111.5605, 7.2485) (-111.5183, 7.127) (-111.4133, 6.9369) (-111.3521, 6.8652) (-111.1527, 6.7072) (-110.9914, 6.6452) (-110.7834, 6.5861) knots -0.259423 -0.259423 -0.259423 -0.259423 -0.144842 -0.144842 -0.103479 -0.103479 -0.064876 -0.064876 0 0 0 0
  spline S4 degree 3 poles (-110.0378, 12.6085) (-110.3914, 12.5916) (-110.6722, 12.5687) (-111.0092, 12.4798) (-111.11, 12.4393) (-111.2822, 12.3287) (-111.3514, 12.261) (-111.4778, 12.0775) (-111.5309, 11.9522) (-111.684, 11.359) (-111.7003, 10.6815) (-111.7005, 9.6175) knots -0.816316 -0.816316 -0.816316 -0.816316 -0.628148 -0.628148 -0.530098 -0.530098 -0.434703 -0.434703 -0.319204 -0.319204 0 0 0 0
  line L30 (-110.0378, 12.6085) -> (-109.2238, 12.6474)
  line L31 (-109.2238, 12.6474) -> (-109.2238, 11.0653)
  line L32 (-109.2238, 11.0653) -> (-110.1412, 11.0653)
  line L33 (-110.1412, 11.0653) -> (-110.1412, 8.0379)
  line L34 (-110.1412, 8.0379) -> (-109.2238, 8.0379)
  line L35 (-109.2238, 8.0379) -> (-109.2238, 6.4783)
  line L36 (-57.8738, 6.4783) -> (-58.6331, 6.4783)
  line L37 (-58.6331, 6.4783) -> (-59.5715, 9.4828)
  spline S5 degree 3 poles (-60.5094, 12.5561) (-60.5096, 12.5287) (-60.2878, 11.8009) (-60.033, 10.9662) (-59.7882, 10.1768) (-59.5715, 9.4828) knots -0.276374 -0.276374 -0.276374 -0.276374 -0.218114 -0.218114 0 0 0 0
  spline S6 degree 3 poles (-59.7363, 12.625) (-60.0215, 12.625) (-60.2722, 12.611) (-60.4322, 12.5864) (-60.4652, 12.5804) (-60.4925, 12.5706) (-60.4983, 12.5681) (-60.5043, 12.5641) (-60.506, 12.5628) (-60.508, 12.5605) (-60.5086, 12.5595) (-60.5092, 12.5578) (-60.5094, 12.557) (-60.5094, 12.5561) knots -0.039663 -0.039663 -0.039663 -0.039663 -0.008749 -0.008749 -0.002732 -0.002732 -0.001169 -0.001169 -0.000569 -0.000569 -0.000248 -0.000248 0 0 0 0
  line L38 (-59.7363, 12.625) -> (-58.9636, 12.625)
  line L39 (-58.9636, 12.625) -> (-58.8693, 12.3268)
  spline S7 degree 3 poles (-57.8738, 6.4783) (-57.7097, 6.4783) (-57.5702, 6.4575) (-57.4211, 6.4558) (-57.3833, 6.458) (-57.3302, 6.471) (-57.3109, 6.4782) (-57.2768, 6.4998) (-57.2631, 6.513) (-57.2388, 6.5481) (-57.2287, 6.5716) (-57.2044, 6.6748) (-57.2081, 6.7844) (-57.3449, 7.5881) (-57.8331, 9.0503) (-58.8693, 12.3268) knots -2.120669 -2.120669 -2.120669 -2.120669 -1.721297 -1.721297 -1.569733 -1.569733 -1.478196 -1.478196 -1.390956 -1.390956 -1.288669 -1.288669 -1.030946 -1.030946 0 0 0 0
  spline S8 degree 3 poles (-62.4093, 6.5979) (-62.4113, 6.5926) (-62.4131, 6.587) (-62.4152, 6.5765) (-62.4157, 6.5714) (-62.4151, 6.561) (-62.4139, 6.5559) (-62.4092, 6.5454) (-62.4055, 6.5406) (-62.3949, 6.5306) (-62.3867, 6.5254) (-62.3564, 6.5122) (-62.3289, 6.5056) (-62.1795, 6.4858) (-61.9801, 6.4866) (-61.6515, 6.4975) knots -0.195528 -0.195528 -0.195528 -0.195528 -0.183541 -0.183541 -0.173019 -0.173019 -0.161744 -0.161744 -0.148939 -0.148939 -0.131274 -0.131274 -0.098644 -0.098644 0 0 0 0
  line L40 (-62.4093, 6.5979) -> (-62.4093, 6.5979)
  spline S9 degree 3 poles (-61.6049, 9.1475) (-61.8438, 8.3817) (-62.1939, 7.2636) (-62.373, 6.7067) (-62.4022, 6.6164) (-62.4093, 6.5979) knots -0.060742 -0.060742 -0.060742 -0.060742 -0.005934 -0.005934 0 0 0 0
  ellipse E0 centre (-61.5196, 9.2955) end of major axis (-60.7852, 11.6422) minor radius 0.0373 (-60.7866, 11.6414) -> (-61.6049, 9.1475) ccw
  spline S10 degree 3 poles (-60.191, 9.8983) (-60.3924, 10.5844) (-60.5821, 11.1698) (-60.7118, 11.5066) (-60.7414, 11.5805) (-60.7668, 11.6253) (-60.7715, 11.6327) (-60.7772, 11.6391) (-60.7787, 11.6406) (-60.7809, 11.642) (-60.7817, 11.6424) (-60.7829, 11.6428) (-60.7834, 11.6428) (-60.7844, 11.6428) (-60.7849, 11.6427) (-60.7858, 11.6422) (-60.7862, 11.6418) (-60.7866, 11.6414) knots -0.066513 -0.066513 -0.066513 -0.066513 -0.012559 -0.012559 -0.002973 -0.002973 -0.001256 -0.001256 -0.000709 -0.000709 -0.000463 -0.000463 -0.00031 -0.00031 -0.00017 -0.00017 0 0 0 0
  spline S11 degree 3 poles (-59.615, 7.9691) (-59.6322, 8.0148) (-59.769, 8.4727) (-59.9235, 8.9902) (-60.0653, 9.4704) (-60.191, 9.8983) knots -0.170058 -0.170058 -0.170058 -0.170058 -0.133786 -0.133786 0 0 0 0
  spline S12 degree 3 poles (-59.9869, 7.8544) (-59.8772, 7.8544) (-59.7735, 7.8589) (-59.6825, 7.8797) (-59.6623, 7.886) (-59.6381, 7.899) (-59.6303, 7.9042) (-59.6198, 7.9152) (-59.6162, 7.9203) (-59.6113, 7.9317) (-59.6101, 7.9377) (-59.61, 7.9525) (-59.612, 7.9611) (-59.615, 7.9691) knots -0.032768 -0.032768 -0.032768 -0.032768 -0.014523 -0.014523 -0.009003 -0.009003 -0.006292 -0.006292 -0.004431 -0.004431 -0.002566 -0.002566 0 0 0 0
  line L41 (-59.9869, 7.8544) -> (-60.4019, 7.8544)
  line L42 (-60.4019, 7.8544) -> (-60.6234, 7.1893)
  line L43 (-60.6234, 7.1893) -> (-60.8449, 6.5241)
  line L44 (-60.8449, 6.5241) -> (-61.6515, 6.4975)
  spline S13 degree 3 poles (-79.849, 59.5684) (-78.209, 60.7567) (-76.7907, 61.7586) (-76.3549, 62.0371) (-76.317, 62.0603) (-76.2944, 62.071) (-76.2907, 62.0726) (-76.2872, 62.0735) (-76.2864, 62.0737) (-76.2858, 62.0737) knots -0.050773 -0.050773 -0.050773 -0.050773 -0.005434 -0.005434 -0.000931 -0.000931 -0.0002 -0.0002 0 0 0 0
  spline S14 degree 3 poles (-84.2701, 56.5783) (-84.2701, 56.559) (-84.2708, 56.5412) (-84.2682, 56.5203) (-84.2669, 56.5145) (-84.2634, 56.5062) (-84.2616, 56.5031) (-84.257, 56.4979) (-84.2543, 56.496) (-84.2471, 56.4926) (-84.2427, 56.4917) (-84.2314, 56.491) (-84.2234, 56.4918) (-84.1516, 56.509) (-84.0219, 56.5831) (-83.2099, 57.1323) (-82.1054, 57.9337) (-79.849, 59.5684) knots -1.606988 -1.606988 -1.606988 -1.606988 -1.483799 -1.483799 -1.430752 -1.430752 -1.396378 -1.396378 -1.363169 -1.363169 -1.319405 -1.319405 -1.253877 -1.253877 -0.835903 -0.835903 0 0 0 0
  spline S15 degree 3 poles (-82.9452, 60.7754) (-83.5924, 58.7743) (-84.1378, 57.0523) (-84.2572, 56.6324) (-84.267, 56.597) (-84.2697, 56.5815) (-84.2701, 56.5795) (-84.2701, 56.5783) knots -0.053073 -0.053073 -0.053073 -0.053073 -0.003796 -0.003796 -0.000379 -0.000379 0 0 0 0
  spline S16 degree 3 poles (-81.4857, 65.3419) (-81.5398, 65.1533) (-81.8906, 64.0552) (-82.2727, 62.8596) (-82.626, 61.7625) (-82.9452, 60.7754) knots -0.392919 -0.392919 -0.392919 -0.392919 -0.31122 -0.31122 0 0 0 0
  line L45 (-81.4857, 65.3419) -> (-81.3511, 65.812)
  line L46 (-81.3511, 65.812) -> (-83.2605, 67.2226)
  spline S17 degree 3 poles (-87.1031, 70.0552) (-86.5114, 69.62) (-85.7897, 69.0883) (-84.5675, 68.1873) (-83.8471, 67.656) (-83.2605, 67.2226) knots -0.438844 -0.438844 -0.438844 -0.438844 -0.218813 -0.218813 0 0 0 0
  spline S18 degree 3 poles (-89.0384, 71.5321) (-89.0384, 71.5318) (-89.0384, 71.5315) (-89.0381, 71.5309) (-89.0379, 71.5305) (-89.0372, 71.5292) (-89.0365, 71.5282) (-89.0337, 71.5247) (-89.0306, 71.5215) (-89.0197, 71.5106) (-89.0074, 71.4997) (-88.9657, 71.4635) (-88.9184, 71.4252) (-88.7627, 71.3006) (-88.5947, 71.1715) (-88.0532, 70.7583) (-87.5482, 70.3826) (-87.1031, 70.0552) knots -0.234771 -0.234771 -0.234771 -0.234771 -0.234683 -0.234683 -0.23457 -0.23457 -0.234247 -0.234247 -0.23321 -0.23321 -0.229532 -0.229532 -0.215884 -0.215884 -0.165785 -0.165785 0 0 0 0
  spline S19 degree 3 poles (-83.4072, 71.7078) (-84.6812, 71.7074) (-86.5657, 71.6988) (-88.1778, 71.6393) (-88.6789, 71.616) (-88.9449, 71.5718) (-88.9841, 71.5641) (-89.0171, 71.5517) (-89.0243, 71.5485) (-89.0319, 71.5432) (-89.0341, 71.5414) (-89.0366, 71.5382) (-89.0374, 71.5369) (-89.0383, 71.5344) (-89.0385, 71.5332) (-89.0384, 71.5321) knots -0.233605 -0.233605 -0.233605 -0.233605 -0.060381 -0.060381 -0.01076 -0.01076 -0.003564 -0.003564 -0.00159 -0.00159 -0.0008 -0.0008 -0.000358 -0.000358 0 0 0 0
  spline S20 degree 3 poles (-79.541, 71.7595) (-79.6159, 71.7394) (-80.5334, 71.7265) (-81.574, 71.7125) (-82.5451, 71.7081) (-83.4072, 71.7078) knots -0.328258 -0.328258 -0.328258 -0.328258 -0.258609 -0.258609 0 0 0 0
  spline S21 degree 3 poles (-77.9172, 76.1848) (-78.8088, 73.4686) (-79.1835, 72.3728) (-79.4184, 71.895) (-79.4492, 71.8434) (-79.4908, 71.7922) (-79.5036, 71.78) (-79.5235, 71.7663) (-79.5319, 71.7619) (-79.541, 71.7595) knots -0.063276 -0.063276 -0.063276 -0.063276 -0.015931 -0.015931 -0.007242 -0.007242 -0.00282 -0.00282 0 0 0 0
  spline S22 degree 3 poles (-76.1729, 80.8806) (-76.1749, 80.8829) (-76.1771, 80.8852) (-76.1818, 80.8889) (-76.1841, 80.8905) (-76.19, 80.8933) (-76.1936, 80.8942) (-76.2016, 80.8946) (-76.2059, 80.8938) (-76.2168, 80.89) (-76.2232, 80.8859) (-76.2533, 80.8617) (-76.2814, 80.8208) (-76.3862, 80.6281) (-76.4827, 80.3921) (-76.8795, 79.3241) (-77.3269, 77.9833) (-77.9172, 76.1848) knots -0.989061 -0.989061 -0.989061 -0.989061 -0.978598 -0.978598 -0.969157 -0.969157 -0.956826 -0.956826 -0.942261 -0.942261 -0.918357 -0.918357 -0.812883 -0.812883 -0.567887 -0.567887 0 0 0 0
  spline S23 degree 3 poles (-75.6599, 79.3211) (-75.8916, 80.0611) (-76.0998, 80.6978) (-76.1621, 80.8579) (-76.1676, 80.8715) (-76.1716, 80.8787) (-76.1723, 80.8799) (-76.1729, 80.8806) knots -0.028216 -0.028216 -0.028216 -0.028216 -0.002031 -0.002031 -0.000276 -0.000276 0 0 0 0
  spline S24 degree 3 poles (-74.1964, 74.7799) (-74.467, 75.6079) (-74.7677, 76.5351) (-75.2184, 77.9336) (-75.4957, 78.7968) (-75.6599, 79.3211) knots -0.403794 -0.403794 -0.403794 -0.403794 -0.164835 -0.164835 0 0 0 0
  line L47 (-74.1964, 74.7799) -> (-73.207, 71.7524)
  line L48 (-73.207, 71.7524) -> (-68.3792, 71.7064)
  spline S25 degree 3 poles (-63.4883, 71.5973) (-63.4886, 71.5976) (-63.4891, 71.5978) (-63.4902, 71.5984) (-63.4909, 71.5987) (-63.4935, 71.5996) (-63.4959, 71.6001) (-63.5045, 71.6019) (-63.5133, 71.6031) (-63.5435, 71.6068) (-63.5763, 71.6093) (-63.6864, 71.6168) (-63.8084, 71.6221) (-64.2081, 71.6377) (-64.6339, 71.6483) (-66.0024, 71.6788) (-67.2682, 71.6958) (-68.3792, 71.7064) knots -0.471489 -0.471489 -0.471489 -0.471489 -0.471339 -0.471339 -0.471132 -0.471132 -0.470522 -0.470522 -0.468497 -0.468497 -0.461199 -0.461199 -0.433901 -0.433901 -0.333337 -0.333337 0 0 0 0
  spline S26 degree 3 poles (-64.3411, 70.8635) (-64.1568, 70.9985) (-63.9581, 71.1505) (-63.7282, 71.3419) (-63.5876, 71.4606) (-63.5103, 71.5486) (-63.4985, 71.5631) (-63.4896, 71.5791) (-63.4877, 71.5831) (-63.4864, 71.5885) (-63.4861, 71.5903) (-63.4862, 71.593) (-63.4864, 71.594) (-63.4872, 71.5958) (-63.4877, 71.5966) (-63.4883, 71.5973) knots -0.092915 -0.092915 -0.092915 -0.092915 -0.028517 -0.028517 -0.005934 -0.005934 -0.002255 -0.002255 -0.001103 -0.001103 -0.000592 -0.000592 -0.00028 -0.00028 0 0 0 0
  spline S27 degree 3 poles (-68.2156, 68.0369) (-67.4485, 68.5958) (-66.6078, 69.2088) (-65.4752, 70.0351) (-64.6817, 70.6141) (-64.3411, 70.8635) knots -0.375651 -0.375651 -0.375651 -0.375651 -0.126642 -0.126642 0 0 0 0
  spline S28 degree 3 poles (-71.2171, 65.7693) (-71.2164, 65.7713) (-71.2142, 65.7743) (-71.2071, 65.7824) (-71.2018, 65.7877) (-71.183, 65.8057) (-71.1631, 65.823) (-71.0951, 65.881) (-71.0209, 65.9402) (-70.7748, 66.1347) (-70.515, 66.3324) (-69.6759, 66.9664) (-68.9013, 67.5372) (-68.2156, 68.0369) knots -0.364151 -0.364151 -0.364151 -0.364151 -0.362708 -0.362708 -0.360844 -0.360844 -0.354658 -0.354658 -0.332742 -0.332742 -0.254521 -0.254521 0 0 0 0
  spline S29 degree 3 poles (-70.4316, 63.1547) (-70.7965, 64.2572) (-71.0963, 65.2325) (-71.2019, 65.6614) (-71.2145, 65.7175) (-71.2181, 65.754) (-71.2185, 65.7605) (-71.2179, 65.7667) (-71.2176, 65.7681) (-71.2171, 65.7693) knots -0.05542 -0.05542 -0.05542 -0.05542 -0.008305 -0.008305 -0.001625 -0.001625 -0.000382 -0.000382 0 0 0 0
  spline S30 degree 3 poles (-68.36, 56.7181) (-68.4184, 56.9651) (-68.9159, 58.5129) (-69.4611, 60.2068) (-69.97, 61.76) (-70.4316, 63.1547) knots -0.55767 -0.55767 -0.55767 -0.55767 -0.440734 -0.440734 0 0 0 0
  spline S31 degree 3 poles (-72.3936, 59.3233) (-70.2, 57.73) (-69.1725, 56.9832) (-68.5867, 56.6177) (-68.5043, 56.573) (-68.4247, 56.542) (-68.4059, 56.5369) (-68.3833, 56.5342) (-68.3753, 56.534) (-68.3634, 56.5363) (-68.359, 56.5378) (-68.3514, 56.5423) (-68.3483, 56.5451) (-68.3425, 56.5529) (-68.3404, 56.5579) (-68.3367, 56.5716) (-68.336, 56.5818) (-68.3379, 56.6256) (-68.3484, 56.6689) (-68.36, 56.7181) knots -0.157965 -0.157965 -0.157965 -0.157965 -0.066725 -0.066725 -0.043668 -0.043668 -0.034179 -0.034179 -0.029512 -0.029512 -0.026647 -0.026647 -0.023998 -0.023998 -0.020658 -0.020658 -0.015175 -0.015175 0 0 0 0
  spline S32 degree 3 poles (-76.2858, 62.0737) (-76.2848, 62.0737) (-76.2834, 62.0733) (-76.2797, 62.0721) (-76.2774, 62.071) (-76.2691, 62.0671) (-76.2613, 62.0628) (-76.2346, 62.0475) (-76.207, 62.0302) (-76.1148, 61.9712) (-76.0158, 61.9043) (-75.6916, 61.6832) (-75.3525, 61.445) (-74.2638, 60.6756) (-73.2672, 59.9578) (-72.3936, 59.3233) knots -0.45996 -0.45996 -0.45996 -0.45996 -0.459443 -0.459443 -0.458784 -0.458784 -0.456678 -0.456678 -0.449314 -0.449314 -0.422307 -0.422307 -0.323934 -0.323934 0 0 0 0
  line L49 (-108.0999, 6.4942) -> (-108.8568, 6.4594)
  line L50 (-108.8568, 6.4594) -> (-108.8568, 7.2486)
  line L51 (-108.8568, 7.2486) -> (-108.8568, 8.0379)
  line L52 (-108.8568, 8.0379) -> (-107.9394, 8.0379)
  line L53 (-107.9394, 8.0379) -> (-107.9394, 11.0653)
  line L54 (-107.9394, 11.0653) -> (-108.8568, 11.0653)
  line L55 (-108.8568, 11.0653) -> (-108.8568, 12.6432)
  line L56 (-108.8568, 12.6432) -> (-108.0377, 12.6111)
  spline S33 degree 3 poles (-106.4003, 9.4434) (-106.3875, 10.5243) (-106.3959, 11.2314) (-106.5283, 11.8621) (-106.5743, 11.9963) (-106.6827, 12.1942) (-106.743, 12.2715) (-106.9048, 12.4064) (-107.0043, 12.4575) (-107.3503, 12.5704) (-107.6492, 12.5959) (-108.0377, 12.6111) knots -0.489269 -0.489269 -0.489269 -0.489269 -0.298589 -0.298589 -0.230659 -0.230659 -0.176091 -0.176091 -0.116644 -0.116644 0 0 0 0
  spline S34 degree 3 poles (-108.0999, 6.4942) (-107.7216, 6.5116) (-107.4287, 6.5329) (-107.0902, 6.6218) (-106.993, 6.6607) (-106.8266, 6.7674) (-106.7596, 6.8327) (-106.637, 7.0104) (-106.5852, 7.1321) (-106.4329, 7.7134) (-106.413, 8.3835) (-106.4003, 9.4434) knots -0.81753 -0.81753 -0.81753 -0.81753 -0.621796 -0.621796 -0.525679 -0.525679 -0.431891 -0.431891 -0.317982 -0.317982 0 0 0 0
  line L57 (-64.6373, 6.4783) -> (-66.197, 6.4783)
  line L58 (-66.197, 6.4783) -> (-66.197, 12.625)
  line L59 (-66.197, 12.625) -> (-64.6373, 12.625)
  line L60 (-64.6373, 12.625) -> (-64.6373, 6.4783)
  line L61 (-94.0864, 6.4783) -> (-95.7683, 6.4783)
  spline S35 degree 3 poles (-97.5114, 6.5394) (-97.5103, 6.5383) (-97.5085, 6.5373) (-97.5031, 6.5351) (-97.4996, 6.534) (-97.4869, 6.5307) (-97.4745, 6.5286) (-97.4319, 6.5222) (-97.3877, 6.5183) (-97.2407, 6.5067) (-97.0898, 6.5003) (-96.6027, 6.4832) (-96.1599, 6.4783) (-95.7683, 6.4783) knots -0.169373 -0.169373 -0.169373 -0.169373 -0.168582 -0.168582 -0.167589 -0.167589 -0.164504 -0.164504 -0.154023 -0.154023 -0.117465 -0.117465 0 0 0 0
  spline S36 degree 3 poles (-97.5726, 7.3192) (-97.5726, 7.0728) (-97.5619, 6.8431) (-97.5412, 6.6579) (-97.5338, 6.6008) (-97.5215, 6.5589) (-97.5187, 6.5509) (-97.5144, 6.5431) (-97.513, 6.541) (-97.5114, 6.5394) knots -0.047138 -0.047138 -0.047138 -0.047138 -0.011977 -0.011977 -0.002675 -0.002675 -0.000673 -0.000673 0 0 0 0
  line L62 (-97.5726, 7.3192) -> (-97.5726, 8.0379)
  line L63 (-97.5726, 8.0379) -> (-94.0864, 8.0379)
  line L64 (-94.0864, 8.0379) -> (-94.0864, 6.4783)
  line L65 (-102.0791, 9.3313) -> (-102.4626, 8.5011)
  spline S37 degree 3 poles (-104.2491, 10.0989) (-103.6394, 8.9644) (-103.3092, 8.3174) (-103.0584, 7.9535) (-103.0129, 7.8941) (-102.9502, 7.8372) (-102.9311, 7.823) (-102.9, 7.808) (-102.8875, 7.8039) (-102.8629, 7.8012) (-102.8515, 7.8022) (-102.8265, 7.8096) (-102.814, 7.8169) (-102.7783, 7.8449) (-102.7547, 7.8754) (-102.6592, 8.0353) (-102.5824, 8.2417) (-102.4626, 8.5011) knots -0.451813 -0.451813 -0.451813 -0.451813 -0.218533 -0.218533 -0.171337 -0.171337 -0.151307 -0.151307 -0.139091 -0.139091 -0.128166 -0.128166 -0.114778 -0.114778 -0.085732 -0.085732 0 0 0 0
  spline S38 degree 3 poles (-105.5541, 12.576) (-105.5541, 12.575) (-105.5534, 12.5728) (-105.551, 12.5666) (-105.5489, 12.5619) (-105.5417, 12.5458) (-105.5334, 12.5287) (-105.5054, 12.4715) (-105.4736, 12.4091) (-105.3688, 12.2048) (-105.2556, 11.9891) (-104.8905, 11.2961) (-104.5498, 10.6584) (-104.2491, 10.0989) knots -0.270154 -0.270154 -0.270154 -0.270154 -0.269348 -0.269348 -0.268163 -0.268163 -0.263927 -0.263927 -0.248198 -0.248198 -0.19054 -0.19054 0 0 0 0
  spline S39 degree 3 poles (-104.7839, 12.6249) (-105.1068, 12.6249) (-105.3853, 12.6121) (-105.5136, 12.5918) (-105.5311, 12.5885) (-105.5454, 12.5834) (-105.5484, 12.5821) (-105.5515, 12.5801) (-105.5524, 12.5794) (-105.5534, 12.5782) (-105.5537, 12.5777) (-105.554, 12.5768) (-105.5541, 12.5764) (-105.5541, 12.576) knots -0.029375 -0.029375 -0.029375 -0.029375 -0.004532 -0.004532 -0.001407 -0.001407 -0.000598 -0.000598 -0.00029 -0.00029 -0.000126 -0.000126 0 0 0 0
  line L66 (-104.7839, 12.6249) -> (-104.0137, 12.6249)
  line L67 (-104.0137, 12.6249) -> (-103.0464, 10.9781)
  line L68 (-103.0464, 10.9781) -> (-102.0791, 9.3313)
  spline S40 degree 3 poles (-114.0861, 10.8818) (-114.0861, 10.8536) (-114.0844, 10.8296) (-114.0746, 10.7978) (-114.0695, 10.7873) (-114.0544, 10.7675) (-114.0442, 10.7586) (-114.014, 10.741) (-113.9923, 10.7331) (-113.8578, 10.7019) (-113.6602, 10.6983) (-113.2953, 10.6983) knots -0.220989 -0.220989 -0.220989 -0.220989 -0.182797 -0.182797 -0.161264 -0.161264 -0.138269 -0.138269 -0.109471 -0.109471 0 0 0 0
  line L69 (-114.0861, 10.8818) -> (-114.0861, 10.8819)
  spline S41 degree 3 poles (-114.5448, 11.0653) (-114.3964, 11.0653) (-114.293, 11.062) (-114.1941, 11.0434) (-114.1711, 11.0364) (-114.1404, 11.0209) (-114.1289, 11.0131) (-114.1097, 10.9928) (-114.1028, 10.9813) (-114.089, 10.9452) (-114.0861, 10.9168) (-114.0861, 10.8819) knots -0.051982 -0.051982 -0.051982 -0.051982 -0.030986 -0.030986 -0.022285 -0.022285 -0.016362 -0.016362 -0.010469 -0.010469 0 0 0 0
  line L70 (-114.5448, 11.0653) -> (-115.0035, 11.0653)
  line L71 (-115.0035, 11.0653) -> (-115.0035, 12.6249)
  line L72 (-115.0035, 12.6249) -> (-114.2925, 12.6247)
  spline S42 degree 3 poles (-112.5443, 11.25) (-112.5542, 11.3861) (-112.573, 11.525) (-112.6353, 11.7719) (-112.6755, 11.8837) (-112.7966, 12.1063) (-112.8797, 12.2091) (-113.1105, 12.3982) (-113.2573, 12.4682) (-113.6495, 12.5906) (-113.9399, 12.6246) (-114.2925, 12.6247) knots -0.340598 -0.340598 -0.340598 -0.340598 -0.282454 -0.282454 -0.232379 -0.232379 -0.174844 -0.174844 -0.105779 -0.105779 0 0 0 0
  line L73 (-112.5443, 11.25) -> (-112.5044, 10.6983)
  line L74 (-112.5044, 10.6983) -> (-113.2953, 10.6983)
  line L75 (-31.9773, 11.0653) -> (-33.5369, 11.0653)
  line L76 (-33.5369, 11.0653) -> (-33.5369, 12.6249)
  line L77 (-33.5369, 12.6249) -> (-31.9773, 12.6249)
  line L78 (-31.9773, 12.6249) -> (-31.9773, 11.0653)
  line L79 (-48.9495, 6.4783) -> (-50.5091, 6.4783)
  line L80 (-50.5091, 6.4783) -> (-50.5091, 12.625)
  line L81 (-50.5091, 12.625) -> (-48.9495, 12.625)
  line L82 (-48.9495, 12.625) -> (-48.9495, 10.3314)
  line L83 (-48.9495, 10.3314) -> (-46.656, 10.3314)
  line L84 (-46.656, 10.3314) -> (-46.656, 8.7718)
  line L85 (-46.656, 8.7718) -> (-48.9495, 8.7718)
  line L86 (-48.9495, 8.7718) -> (-48.9495, 6.4783)
  line L87 (-35.7387, 11.0653) -> (-37.2983, 11.0653)
  line L88 (-37.2983, 11.0653) -> (-37.2983, 12.6249)
  line L89 (-37.2983, 12.6249) -> (-35.7387, 12.6249)
  line L90 (-35.7387, 12.6249) -> (-35.7387, 11.0653)
  line L91 (-100.2331, 6.4783) -> (-101.7927, 6.4783)
  line L92 (-101.7927, 6.4783) -> (-101.7927, 9.6669)